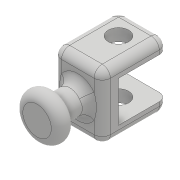
# Autodesk Inventor part: Elo-Bola Longo
Saved by Autodesk Inventor 2018 (Build 220112000, 112)
## iProperties
Created: 2021-04-27
Part Number: Elo-Bola Longo
Material: Generic
Document SubType Name: Modeling
Designer: l01767
Density: 1 g/cm^3
Appearance: Default
Author: l01767
Autodesk Inventor part; units mm, degrees
ref_plane "YZ Plane" through (0, 0, 0) normal (1, 0, 0) x (0, 1, 0)
ref_plane "XZ Plane" through (0, 0, 0) normal (0, 1, 0) x (-1, 0, 0)
ref_plane "XY Plane" through (0, 0, 0) normal (0, 0, 1) x (1, 0, 0)
sketch "Sketch1" plane through (0, 0, 0) normal (0, 0, 1) x (1, 0, 0)
  line L0 (0, 0) -> (0, 40)
  dimension "d0" = 40
  constraints: 2 end point, 1 vertical
  measures "d0" distance of L0.start L0.end
sketch "Sketch2" plane through (0, 0, 0) normal (0, 1, 0) x (-1, 0, 0)
  circle A0 centre (0, 0) radius 15
  dimension "d3" = 30
  constraints: 1 centre point, 1 coincident
  measures "d3" diameter of A0
sweep "Sweep1" add profiles "Sketch2" path "Sketch1"
sketch "Sketch4" plane through (0, 0, 0) normal (1, 0, 0) x (0, 1, 0)
  line L0 (0, 17.5) -> (0, -17.5) construction
  line L1 (10, 17.5) -> (10, -17.5)
  line L2 (-10, -17.5) -> (-10, 17.5)
  arc A0 (10, 17.5) -> (-10, 17.5) centre (0, 17.5) ccw
  arc A1 (-10, -17.5) -> (10, -17.5) centre (0, -17.5) ccw
  line L3 (-10, 0) -> (10, 0)
  point P0 (0, 0)
  dimension "d9" = 35
  dimension "d10" = 10
  constraints: 10 end point, 4 point on circle, 4 tangent, 3 midpoint, 2 centre point, 1 parallel, 1 vertical
  measures "d9" distance of L0.start L0.end
  measures "d10" radius of A1
revolve "Revolution1" add sketch "Sketch4" angle 360 about axis through (0, -10, 0) along (0, 1, 0) contours L1 L3 L2 A0
sketch "Sketch5" plane through (0, 0, 0) normal (0, 0, 1) x (1, 0, 0)
  line L0 (-30, 40) -> (30, 40)
  line L1 (30, 40) -> (30, 120)
  line L2 (30, 120) -> (-30, 120)
  line L3 (-30, 120) -> (-30, 40)
  circle A0 centre (0, 90) radius 12.5
  line L4 (0, 0) -> (0, 40) construction
  line L5 (0, 90) -> (0, 40)
  dimension "d12" = 90
  dimension "d13" = 25
  dimension "d14" = 60
  dimension "d15" = 30
  constraints: 10 end point, 2 parallel, 1 centre point, 1 horizontal, 1 midpoint, 1 perpendicular, 1 vertical, 1 other
  measures "d12" distance of point (0, 0) L5.start
  measures "d13" diameter of A0
  measures "d14" distance of L1.end L2.end
  measures "d15" distance from line of L5.start L2
extrude "Extrusion1" add sketch "Sketch5" along normal mid plane 80
sketch "Sketch7" plane through (-30, 40, 40) normal (-1, 0, 0) x (0, 0, 1)
  line L0 (-80, 80) -> (0, 80) construction
  line L1 (-65, 80) -> (-15, 80)
  line L2 (-15, 80) -> (-15, 20)
  line L3 (-15, 20) -> (-65, 20)
  line L4 (-65, 20) -> (-65, 80)
  line L5 (-80, 37.5) -> (-80, 62.5) construction
  line L6 (0, 62.5) -> (0, 37.5) construction
  line L7 (-80, 0) -> (-80, 80) construction
  line L8 (-80, 50) -> (0, 50) construction
  line L9 (0, 80) -> (0, 0) construction
  line L10 (-40, 50) -> (-40, 0) construction
  point P0 (-40, -40)
  dimension "d18" = 30
  dimension "d19" = 50
  dimension "d20" = 25
  dimension "d21" = 90
  constraints: 12 end point, 3 point on line, 2 parallel, 2 perpendicular, 1 horizontal, 1 midpoint, 1 vertical
  measures "d18" distance between parallel lines of L3 L8
  measures "d19" distance of L1.start L1.end
  measures "d20" distance between parallel lines of L4 L10
  measures "d21" distance from line of point (-40, -40) L8
fillet "Fillet1" radius 10 13 edges at (-30, 80, 40) (30, 80, 40) (-30, 80, -40) (30, 80, -40) (-30, 40, 0) (0, 40, -40) (0, 40, 40) (30, 40, 0) (15, 40, 0) (-30, 120, 0) (0, 120, 40) (30, 120, 0) (0, 120, -40)
extrude "Extrusion2" cut sketch "Sketch7" against normal through all
equation "\"d20\" = 0.5 * d19"
body "Solid1"
